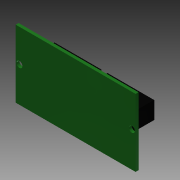
# Autodesk Inventor part: powerdistv2
Saved by Autodesk Inventor 2015 (Build 190159000, 159)
## iProperties
Created: 2015-02-04
Part Number: powerdistv2
Material: Generic
Document SubType Name: Modeling
Designer: Rafi Kurnia Putra
Density: 1 g/cm^3
Appearance: Smooth - Dark Forest Green
Mass: 12.5901 g
Surface Area: 79.6628 cm^2
Volume: 12.5901 cm^3
Author: Rafi Kurnia Putra
Autodesk Inventor part; units mm, degrees
ref_plane "YZ Plane" through (0, 0, 0) normal (1, 0, 0) x (0, 1, 0)
ref_plane "XZ Plane" through (0, 0, 0) normal (0, 1, 0) x (-1, 0, 0)
ref_plane "XY Plane" through (0, 0, 0) normal (0, 0, 1) x (1, 0, 0)
sketch "Sketch1" plane through (0, 0, 0) normal (0, 1, 0) x (-1, 0, 0)
  line L0 (34.6075, 19.4945) -> (-34.6075, 19.4945)
  line L1 (-34.6075, 19.4945) -> (-34.6075, -19.4945)
  line L2 (-34.6075, -19.4945) -> (34.6075, -19.4945)
  line L3 (34.6075, -19.4945) -> (34.6075, 19.4945)
  line L4 (-34.6075, 19.4945) -> (34.6075, -19.4945) construction
  circle A0 centre (32.4355, 0.7215) radius 1.75
  circle A1 centre (-32.4485, 0.7215) radius 1.75
  line L5 (28.7695, 5.2375) -> (1.7695, 5.2375)
  line L6 (1.7695, 5.2375) -> (1.7695, -4.7625)
  line L7 (1.7695, -4.7625) -> (28.7695, -4.7625)
  line L8 (28.7695, -4.7625) -> (28.7695, 5.2375)
  line L9 (28.7695, 5.2375) -> (1.7695, -4.7625) construction
  line L10 (1.7695, 5.2375) -> (28.7695, -4.7625) construction
  line L11 (-28.7695, 5.2375) -> (-1.7695, 5.2375)
  line L12 (-1.7695, 5.2375) -> (-1.7695, -4.7625)
  line L13 (-1.7695, -4.7625) -> (-28.7695, -4.7625)
  line L14 (-28.7695, -4.7625) -> (-28.7695, 5.2375)
  point P0 (0, 0)
  point P1 (15.2695, 0.2375)
  dimension "d0" = 69.215
  dimension "d1" = 38.989
  dimension "d2" = 3.5
  dimension "d3" = 2.172
  dimension "d4" = 20.216
  dimension "d5" = 27
  dimension "d6" = 10
  dimension "d18" = 64.884
  constraints: 30 end point, 4 parallel, 3 midpoint, 2 centre point, 2 horizontal, 2 perpendicular
  measures "d0" distance of L2.end L1.end
  measures "d1" distance of L1.end L0.end
  measures "d2" diameter of A0
  measures "d3" distance from line of A0.centre L3
  measures "d4" distance from line of L2 A0.centre
  measures "d5" distance of L7.end L6.end
  measures "d6" distance of L6.end L5.end
  measures "d18" distance of A1.centre A0.centre
extrude "Extrusion1" add sketch "Sketch1" along normal blind 1.7
extrude "Extrusion2" add sketch "Sketch1" along normal blind 16.58 contours L8 L7 L6 L5 | L11 L12 L13 L14
sketch "Sketch2" plane through (0, 1.7, 0) normal (0, 1, 0) x (1, 0, 0)
  line L0 (-16.1466, -9.4421) -> (18.9981, -9.4421) construction
  line L1 (18.9981, -9.4421) -> (18.9981, -13.0896) construction
  line L2 (18.9981, -13.0896) -> (-16.1466, -13.0896) construction
  line L3 (-16.1466, -13.0896) -> (-16.1466, -9.4421) construction
  point P0 (0, 0)
  constraints: 2 other
body "Solid1"
